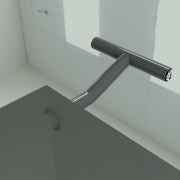
# Autodesk Inventor part: Bootsklampe Metall
Saved by Autodesk Inventor 2015 (Build 190159000, 159)
## iProperties
Created: 2017-04-12
Part Number: Bootsklampe Metall
Material: Generic
Document SubType Name: Modeling
Designer: Seelenernter
Density: 1 g/cm^3
Appearance: Galvanisiert
Author: Seelenernter
Autodesk Inventor part; units mm, degrees
ref_plane "YZ Plane" through (0, 0, 0) normal (1, 0, 0) x (0, 1, 0)
ref_plane "XZ Plane" through (0, 0, 0) normal (0, 1, 0) x (-1, 0, 0)
sketch "Skizze1" plane through (0, 0, 0) normal (0, 1, 0) x (-1, 0, 0)
  circle A0 centre (0, 0) radius 15
  dimension "d0" = 30
  constraints: 1 centre point, 1 coincident
  measures "d0" diameter of A0
sketch "Skizze2" plane through (0, 0, 0) normal (1, 0, 0) x (0, 1, 0)
  line L0 (0, 0) -> (122.9469, 0)
  line L1 (136.6277, 2.4123) -> (252.16, 44.4626)
  arc A0 (122.9469, 0) -> (136.6277, 2.4123) centre (122.9469, 40) ccw
  point P0 (130, 0)
  dimension "d1" = 160
  dimension "d2" = 130
  dimension "d3" = 130
  dimension "d4" = 40
  constraints: 4 end point, 2 point on circle, 2 point on line, 2 tangent, 1 centre point, 1 horizontal
  measures "d1" angle of L0 L1
  measures "d2" distance of point (130, 0) L1.end
  measures "d3" distance of L0.start point (130, 0)
  measures "d4" radius of A0
sweep "Sweeping1" add profiles "Skizze1" path "Skizze2"
sketch "Skizze3" plane through (0, 0, 0) normal (1, 0, 0) x (0, 1, 0)
  line L0 (257.2903, 30.3672) -> (247.0297, 58.558) projected
  line L1 (141.758, -11.6831) -> (131.4974, 16.5077) projected
  line L2 (257.2903, 30.3672) -> (247.0297, 58.558) projected
  circle A0 centre (252.16, 44.4626) radius 15
  point P0 (0, 0)
  constraints: 1 midpoint, 3 other
extrude "Extrusion1" add sketch "Skizze3" along normal mid plane 200
ref_plane "Arbeitsebene1" through (0, 40, 0) normal (0, -1, 0) x (1, 0, 0)
sketch "Skizze4" plane through (0, 40, 0) normal (0, -1, 0) x (1, 0, 0)
  circle A0 centre (0, 0) radius 25
  dimension "d10" = 50
  constraints: 1 centre point, 1 coincident
  measures "d10" diameter of A0
extrude "Extrusion2" add sketch "Skizze4" along normal blind 3
sketch "Skizze5" plane through (100, 252.16, 44.4626) normal (1, 0, 0) x (0, 0, -1)
  circle A0 centre (0, 0) radius 14
  point P0 (44.4626, -252.16)
  dimension "d13" = 28
  constraints: 1 centre point
  measures "d13" diameter of A0
extrude "Extrusion3" add sketch "Skizze5" along normal blind 2
sketch "Skizze6" plane through (-100, 252.16, 44.4626) normal (-1, 0, 0) x (0, 0, 1)
  circle A0 centre (0, 0) radius 14
  point P0 (-44.4626, -252.16)
  dimension "d16" = 28
  constraints: 1 centre point
  measures "d16" diameter of A0
extrude "Extrusion4" add sketch "Skizze6" along normal blind 2
chamfer "Fase1" distance 1 angle 45 2 edges at (102, 252.16, 58.4626) (-102, 252.16, 30.4626)
